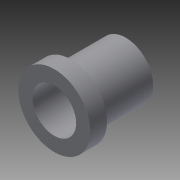
# Autodesk Inventor part: Big Bearing Sleeve
Saved by Autodesk Inventor 2014 (Build 180170000, 170)
## iProperties
Created: 2015-02-12
Part Number: Big Bearing Sleeve
Material: Generic
Document SubType Name: Modeling
Designer: Spooner
Density: 1 g/cm^3
Appearance: Default
Author: Spooner
Autodesk Inventor part; units mm, degrees
ref_plane "YZ Plane" through (0, 0, 0) normal (1, 0, 0) x (0, 1, 0)
ref_plane "XZ Plane" through (0, 0, 0) normal (0, 1, 0) x (-1, 0, 0)
ref_plane "XY Plane" through (0, 0, 0) normal (0, 0, 1) x (1, 0, 0)
ref_plane "Work Plane1" through (0, 0, 0) normal (0, 0, 1) x (1, 0, 0)
sketch "Sketch1" plane through (0, 0, 0) normal (0, 0, 1) x (1, 0, 0)
  circle A0 centre (0, 0) radius 8.5725 projected
  circle A1 centre (0, 0) radius 8.3185
  circle A2 centre (0, 0) radius 6.604
  point P0 (0, 0)
  dimension "d0" = 0.254
  dimension "d1" = 13.208
  constraints: 2 centre point, 2 coincident
  measures "d0" radial gap between concentric circles of A0 A1
  measures "d1" diameter of A2
ref_plane "Work Plane2" through (-23.495, -23.495, -13.97) normal (0, 0, -1) x (0, 1, 0)
extrude "Extrusion1" add sketch "Sketch1" against normal up to surface (13.97 mm away) contours A1
sketch "Sketch2" plane through (0, 0, 0) normal (0, 0, 1) x (1, 0, 0)
  circle A0 centre (0, 0) radius 6.604 projected
  circle A1 centre (0, 0) radius 8.3185 projected
  circle A2 centre (0, 0) radius 10.8585
  dimension "d4" = 2.54
  constraints: 1 centre point, 1 coincident
  measures "d4" radial gap between concentric circles of A1 A2
extrude "Extrusion2" add sketch "Sketch2" along normal blind 5.08 contours A1 | A2
sketch "Sketch4" plane through (0, 0, -13.97) normal (0, 0, -1) x (-1, 0, 0)
  circle A0 centre (0, 0) radius 6.604 projected
  circle A1 centre (0, 0) radius 8.3185 projected
  circle A2 centre (0, 0) radius 4.064
  dimension "d9" = 2.54
  constraints: 1 centre point, 1 coincident
  measures "d9" radial gap between concentric circles of A0 A2
extrude "Extrusion4" add sketch "Sketch4" along normal blind 2.54 contours A0 | A1
body "Solid1"
